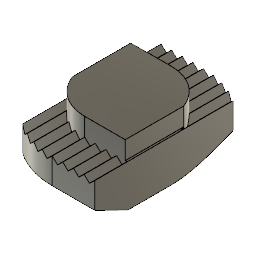
T-Slot_Nut_DropIn_Blank v2 (Autodesk Fusion 360 design; units mm, degrees)
Autodesk Fusion 360 part; units mm, degrees
note: some values were not read from the file. Chosen so that the rebuilt part matches the saved one: where a step starts.
sketch "Sketch1" plane through (0, 0, 0) normal (0, 0, 1) x (1, 0, 0)
  line L0 (2.95, -5.25) -> (-2.95, -5.25)
  line L1 (-2.95, -5.25) -> (-2.95, 5.25)
  line L2 (-2.95, 5.25) -> (2.95, 5.25)
  line L3 (2.95, 5.25) -> (2.95, -5.25)
  line L4 (2.95, -5.25) -> (-2.95, 5.25) construction
  line L5 (-2.95, -5.25) -> (2.95, 5.25) construction
  dimension "d1" = 5.9
  dimension "d2" = 10.5
extrude "Extrude1" add sketch "Sketch1" along normal blind 4.4
sketch "Sketch2" plane through (0, 0, 0) normal (0, 0, -1) x (1, 0, 0)
  line L0 (-2.95, -5.25) -> (2.95, -5.25)
  line L1 (2.95, -5.25) -> (2.95, 5.25)
  line L2 (2.95, 5.25) -> (-2.95, 5.25)
  line L3 (-2.95, 5.25) -> (-2.95, -5.25)
  line L4 (2.95, 2.5) -> (-2.95, 2.5)
  line L5 (-2.95, 2.5) -> (-2.95, -2.5)
  line L6 (-2.95, -2.5) -> (2.95, -2.5)
  line L7 (2.95, -2.5) -> (2.95, 2.5)
  line L8 (2.95, 2.5) -> (-2.95, -2.5) construction
  line L9 (-2.95, 2.5) -> (2.95, -2.5) construction
  dimension "d5" = 5.9
  dimension "d6" = 5
chamfer "Chamfer1" distance 2.75 distance2 1.35 2 edges at (0, -5.25, 0) (0, 5.25, 0) measured on face at (-0.9833, 1.75, 0) measured on face at (-0.9833, 1.75, 0)
sketch "Sketch3" plane through (0, 0, 4.4) normal (0, 0, 1) x (-1, 0, 0)
  line L0 (-2.95, -5.25) -> (2.95, -5.25)
  line L1 (2.95, -5.25) -> (2.95, 5.25)
  line L2 (2.95, 5.25) -> (-2.95, 5.25)
  line L3 (-2.95, 5.25) -> (-2.95, -5.25)
  line L4 (-2.95, 3) -> (2.95, 3)
  line L5 (2.95, 3) -> (2.95, -3)
  line L6 (2.95, -3) -> (-2.95, -3)
  line L7 (-2.95, -3) -> (-2.95, 3)
  line L8 (-2.95, 3) -> (2.95, -3) construction
  line L9 (2.95, 3) -> (-2.95, -3) construction
  circle A0 centre (0, 0) radius 3
  dimension "d9" = 5.9
  dimension "d10" = 6
extrude "Extrude2" cut sketch "Sketch3" against normal blind 1.25 contours L0 L1 L3 L6 | L3 L6 L7 A0 | L1 L4 L5 A0 | L1 L2 L3 L4
ref_plane "WorkPlane1" through (0, 0, 2.2) normal (-1, 0, 0) x (0, -1, 0)
sketch "Sketch4" plane through (0, 0, 2.2) normal (-1, 0, 0) x (0, 1, 0)
  line L0 (-5.25, -0.95) -> (5.25, -0.95)
  line L1 (5.25, -0.95) -> (5.25, 0.85)
  line L2 (5.25, 0.85) -> (-5.25, 0.85)
  line L3 (-5.25, 0.85) -> (-5.25, -0.95)
  line L4 (-5.25, -0.95) -> (5.25, -0.95)
  line L5 (5.25, -0.95) -> (5.25, 2.2)
  line L6 (5.25, 2.2) -> (-5.25, 2.2)
  line L7 (-5.25, 2.2) -> (-5.25, -0.95)
  line L8 (2.5, 2.2) -> (5.25, 0.85)
  line L9 (5.25, 0.85) -> (2.5, 2.2)
  line L10 (-5.25, 0.85) -> (-2.5, 2.2)
  line L11 (-5.25, 0.85) -> (-2.5, 2.2)
  line L12 (-3, -2.2) -> (0.5454, -2.2)
  line L13 (0, 2.2) -> (0, -2.2) construction
  line L14 (-6.4, 2.2) -> (6.4, 2.2)
  line L15 (6.4, 2.2) -> (6.4, -2.2)
  line L16 (6.4, -2.2) -> (-6.4, -2.2)
  line L17 (-6.4, -2.2) -> (-6.4, 2.2)
  line L18 (-6.4, 2.2) -> (6.4, -2.2) construction
  line L19 (6.4, 2.2) -> (-6.4, -2.2) construction
  line L20 (-6.4, -0.95) -> (6.4, -0.95)
  line L21 (6.4, -0.95) -> (6.4, -2.2)
  line L22 (6.4, -2.2) -> (-6.4, -2.2)
  line L23 (-6.4, -2.2) -> (-6.4, -0.95)
sketch "Sketch5" plane through (0, 0, 0) normal (0, 0, -1) x (1, 0, 0)
  line L0 (-2.95, -2.5) -> (2.95, -2.5)
  line L1 (2.95, -2.5) -> (2.95, 2.5)
  line L2 (2.95, 2.5) -> (-2.95, 2.5)
  line L3 (-2.95, 2.5) -> (-2.95, -2.5)
  circle A0 centre (0, 0) radius 6.022
sweep "Sweep1" cut profiles "Sketch4" path "Sketch5" along A0 for 0.25 of its length starting at (6.022, 0, 0) heading (0, 1, 0) section 1 contours L3 L7 L14 L17 L20 | L6 L7 L10 L11 L14
sweep "Sweep2" cut profiles "Sketch4" path "Sketch5" along A0 for 0.25 of its length starting at (6.022, 0, 0) heading (0, 1, 0) section 1 contours L1 L5 L14 L15 L20 | L5 L6 L8 L9 L14
extrude "Extrude3" cut 1 faces at (-2.8, 0, 0.0736) along direction (0, 1, 0) blind 3
extrude "Extrude4" cut 1 faces at (2.8, 0, 0.0736) along direction (0, -1, 0) blind 3
sketch "Sketch6" plane through (0, 0, 4.4) normal (0, 0, 1) x (-1, 0, 0)
  arc A0 (2.95, 0.5454) -> (0, 3) centre (0, 0) ccw
  line L0 (0, 3) -> (-2.95, 3)
  line L1 (-2.95, 3) -> (-2.95, -0.5454)
  arc A1 (-2.95, -0.5454) -> (0, -3) centre (0, 0) ccw
  line L2 (0, -3) -> (2.95, -3)
  line L3 (2.95, -3) -> (2.95, 0.5454)
  line L4 (2.81, -3) -> (-2.81, -3)
  line L5 (-2.81, -3) -> (-2.81, 3)
  line L6 (-2.81, 3) -> (2.81, 3)
  line L7 (2.81, 3) -> (2.81, -3)
  line L8 (2.81, -3) -> (-2.81, 3) construction
  line L9 (-2.81, -3) -> (2.81, 3) construction
  dimension "d29" = 5.62
  dimension "d30" = 6
extrude "Extrude5" cut sketch "Sketch6" against normal blind 1.25 contours A0 L2 L3 L7 | L0 L1 A1 L5
sketch "Sketch7" plane through (0, 0, 3.15) normal (0, 0, 1) x (-1, 0, 0)
  line L0 (-2.81, 3) -> (0, 3)
  arc A0 (2.81, 1.0507) -> (0, 3) centre (0, 0) ccw
  line L1 (2.81, 1.0507) -> (2.81, -3)
  line L2 (2.81, -3) -> (0, -3)
  arc A1 (-2.81, -1.0507) -> (0, -3) centre (0, 0) ccw
  line L3 (-2.81, -1.0507) -> (-2.81, 3)
  line L4 (-2.95, 5.25) -> (-2.95, -4.3428)
  arc A2 (-2.95, -4.3428) -> (0, -5.25) centre (0, 0) ccw
  line L5 (0, -5.25) -> (2.95, -5.25)
  line L6 (2.95, -5.25) -> (2.95, 4.3428)
  arc A3 (2.95, 4.3428) -> (0, 5.25) centre (0, 0) ccw
  line L7 (0, 5.25) -> (-2.95, 5.25)
  line L8 (2.95, -5.25) -> (-2.95, -5.25)
  line L9 (-2.95, -5.25) -> (-2.95, 5.25)
  line L10 (-2.95, 5.25) -> (2.95, 5.25)
  line L11 (2.95, 5.25) -> (2.95, -5.25)
  line L12 (-2.95, 5.25) -> (-2.2125, 5.25)
  line L13 (-2.2125, 5.25) -> (-1.475, 5.25)
  line L14 (-1.475, 5.25) -> (-0.7375, 5.25)
  line L15 (-0.7375, 5.25) -> (0, 5.25)
  line L16 (0, 5.25) -> (0.7375, 5.25)
  line L17 (0.7375, 5.25) -> (1.475, 5.25)
  line L18 (1.475, 5.25) -> (2.2125, 5.25)
  line L19 (2.2125, 5.25) -> (2.95, 5.25)
  line L20 (-2.2125, 5.25) -> (-2.2125, -5.25)
  line L21 (-1.475, 5.25) -> (-1.475, -5.25)
  line L22 (-0.7375, 5.25) -> (-0.7375, -5.25)
  line L23 (0, 5.25) -> (0, -5.25)
  line L24 (0.7375, 5.25) -> (0.7375, -5.25)
  line L25 (1.475, 5.25) -> (1.475, -5.25)
  line L26 (2.2125, 5.25) -> (2.2125, -5.25)
  dimension "d33" = 0.7375
  dimension "d34" = 0.7375
  dimension "d35" = 0.7375
  dimension "d36" = 0.7375
  dimension "d37" = 0.7375
  dimension "d38" = 0.7375
  dimension "d39" = 0.7375
ref_plane "WorkPlane2" through (-1.475, 0, 2.25) normal (0, 1, 0) x (-1, 0, 0)
sketch "Sketch8" plane through (-1.475, 0, 2.25) normal (0, 1, 0) x (1, 0, 0)
  line L0 (-1.475, -0.9) -> (4.425, -0.9)
  line L1 (4.425, -0.9) -> (4.425, -0.55)
  line L2 (4.425, -0.55) -> (-1.475, -0.55)
  line L3 (-1.475, -0.55) -> (-1.475, -0.9)
  line L4 (4.425, 0.9) -> (4.425, -0.9)
  line L5 (-0.7375, -0.9, -5.25) -> (-0.7375, -0.9, 5.25)
  line L6 (-1.475, -0.9) -> (-0.7375, -0.9)
  line L7 (0, -0.9, -5.25) -> (0, -0.9, 5.25)
  line L8 (-0.7375, -0.9) -> (0, -0.9)
  line L9 (0.7375, -0.9, -5.25) -> (0.7375, -0.9, 5.25)
  line L10 (0, -0.9) -> (0.7375, -0.9)
  line L11 (0.7375, -0.9) -> (1.475, -0.9)
  line L12 (2.2125, -0.9, -5.25) -> (2.2125, -0.9, 5.25)
  line L13 (1.475, -0.9) -> (2.2125, -0.9)
  line L14 (2.95, -0.9, -5.25) -> (2.95, -0.9, 5.25)
  line L15 (2.2125, -0.9) -> (2.95, -0.9)
  line L16 (3.6875, -0.9, -5.25) -> (3.6875, -0.9, 5.25)
  line L17 (2.95, -0.9) -> (3.6875, -0.9)
  line L18 (3.6875, -0.9) -> (4.425, -0.9)
  line L19 (4.0563, -0.9) -> (4.0563, -0.55) construction
  line L20 (3.3188, -0.9) -> (3.3188, -0.55) construction
  line L21 (2.5812, -0.9) -> (2.5812, -0.55) construction
  line L22 (1.8438, -0.9) -> (1.8438, -0.55) construction
  line L23 (1.1062, -0.9) -> (1.1062, -0.55) construction
  line L24 (0.3687, -0.9) -> (0.3687, -0.55) construction
  line L25 (-0.3688, -0.9) -> (-0.3688, -0.55) construction
  line L26 (-1.1063, -0.9) -> (-1.1063, -0.55) construction
  line L27 (-1.475, -0.9) -> (-1.1063, -0.55)
  line L28 (-1.1063, -0.55) -> (-0.7375, -0.9)
  line L29 (-0.7375, -0.9) -> (-0.3688, -0.55)
  line L30 (-0.3688, -0.55) -> (0, -0.9)
  line L31 (0, -0.9) -> (0.3687, -0.55)
  line L32 (0.3687, -0.55) -> (0.7375, -0.9)
  line L33 (0.7375, -0.9) -> (1.1062, -0.55)
  line L34 (1.1062, -0.55) -> (1.475, -0.9)
  line L35 (1.475, -0.9) -> (1.8438, -0.55)
  line L36 (1.8438, -0.55) -> (2.2125, -0.9)
  line L37 (2.2125, -0.9) -> (2.5813, -0.55)
  line L38 (2.5812, -0.55) -> (2.95, -0.9)
  line L39 (2.95, -0.9) -> (3.3188, -0.55)
  line L40 (3.3188, -0.55) -> (3.6875, -0.9)
  line L41 (3.6875, -0.9) -> (4.0563, -0.55)
  line L42 (4.0563, -0.55) -> (4.425, -0.9)
  dimension "d40" = 0.35
sketch "Sketch9" plane through (0, 0, 3.15) normal (0, 0, 1) x (-1, 0, 0)
  line L0 (-2.81, 3) -> (0, 3)
  arc A0 (2.81, 1.0507) -> (0, 3) centre (0, 0) ccw
  line L1 (2.81, 1.0507) -> (2.81, -3)
  line L2 (2.81, -3) -> (0, -3)
  arc A1 (-2.81, -1.0507) -> (0, -3) centre (0, 0) ccw
  line L3 (-2.81, -1.0507) -> (-2.81, 3)
  line L4 (-2.95, 5.25) -> (-2.95, -4.3428)
  arc A2 (-2.95, -4.3428) -> (0, -5.25) centre (0, 0) ccw
  line L5 (0, -5.25) -> (2.95, -5.25)
  line L6 (2.95, -5.25) -> (2.95, 4.3428)
  arc A3 (2.95, 4.3428) -> (0, 5.25) centre (0, 0) ccw
  line L7 (0, 5.25) -> (-2.95, 5.25)
  line L8 (2.83, -5.13) -> (2.83, 4.2788)
  arc A4 (2.83, 4.2788) -> (0, 5.13) centre (0, 0) ccw
  line L9 (0, 5.13) -> (-2.83, 5.13)
  line L10 (-2.83, 5.13) -> (-2.83, -4.2788)
  arc A5 (-2.83, -4.2788) -> (0, -5.13) centre (0, 0) ccw
  line L11 (0, -5.13) -> (2.83, -5.13)
  line L12 (2.81, -3) -> (0, -3)
  arc A6 (-2.81, -1.0507) -> (0, -3) centre (0, 0) ccw
  line L13 (-2.81, -1.0507) -> (-2.81, 3)
  line L14 (-2.81, 3) -> (0, 3)
  arc A7 (2.81, 1.0507) -> (0, 3) centre (0, 0) ccw
  line L15 (2.81, 1.0507) -> (2.81, -3)
  line L16 (-2.81, 3) -> (-2.95, 3)
  line L17 (-2.83, 5.13) -> (-2.95, 5.13)
  line L18 (2.83, 4.2788) -> (2.95, 4.1994)
  line L19 (2.81, 1.0507) -> (2.95, 0.6762)
  line L20 (2.81, -3) -> (2.95, -3)
  line L21 (-2.81, -1.0507) -> (-2.95, -0.6762)
  line L22 (-2.83, -4.2788) -> (-2.95, -4.1994)
  line L23 (2.83, -5.13) -> (2.95, -5.13)
  dimension "d41" = 0.12
  dimension "d42" = 0
  measures "d41" distance of L6
  measures "d42" distance of L2
extrude "Extrude6" cut sketch "Sketch8" along normal mid plane 10.5 contours L0 L6 L27 L28 | L0 L8 L29 L30 | L0 L10 L31 L32 | L0 L11 L33 L34 | L0 L13 L35 L36 | L0 L15 L37 L38 | L0 L17 L39 L40 | L0 L18 L41 L42
extrude "Extrude7" add sketch "Sketch9" against normal blind 0.4 contours L0 A0 L1 L2 A1 L3 L12 A6 L13 L14 A7 L15 | L3 L10 L13 L16 L21 | L4 L10 L16 L21 | L1 L8 L15 L19 L20 | L6 L8 L19 L20
